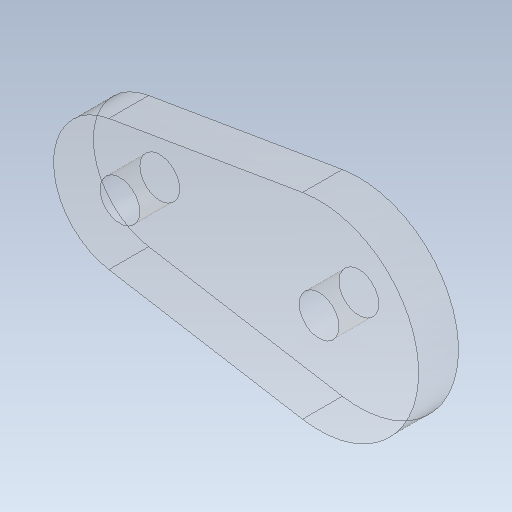
# Autodesk Inventor part: ウイング抑え
Saved by Autodesk Inventor 2020 (Build 240168000, 168)
## iProperties
Created: 2019-11-29
Part Number: ウイング抑え
Material: ポリカーボネート、クリア
Document SubType Name: Modeling
Designer: tanjihayato
Density: 1.2 g/cm^3
Appearance: ポリカーボネート - クリア
Mass: 1.09296 g
Surface Area: 8.72812 cm^2
Volume: 0.910801 cm^3
Author: tanjihayato
Autodesk Inventor part; units mm, degrees
ref_plane "YZ Plane" through (0, 0, 0) normal (1, 0, 0) x (0, 1, 0)
ref_plane "XZ Plane" through (0, 0, 0) normal (0, 1, 0) x (-1, 0, 0)
ref_plane "XY Plane" through (0, 0, 0) normal (0, 0, 1) x (1, 0, 0)
sketch "スケッチ1" plane through (0, 0, 0) normal (0, 0, 1) x (1, 0, 0)
  circle A0 centre (0, 0) radius 1.5
  circle A1 centre (15, 0) radius 1.5
  arc A2 (-0.8333, 4.9301) -> (-0.8333, -4.9301) centre (0, 0) ccw
  arc A3 (13.75, -7.3951) -> (13.75, 7.3951) centre (15, 0) ccw
  line L0 (-0.8333, 4.9301) -> (13.75, 7.3951)
  line L1 (-0.8333, -4.9301) -> (13.75, -7.3951)
  dimension "d0" = 3
  dimension "d1" = 3
  dimension "d2" = 15
  dimension "d3" = 10
  dimension "d4" = 15
  constraints: 4 centre point, 4 end point, 4 point on circle, 4 tangent, 3 coincident, 1 horizontal alignment
  measures "d0" diameter of A0
  measures "d1" diameter of A1
  measures "d2" distance of A1.centre point (0, 0)
  measures "d3" diameter of A2
  measures "d4" diameter of A3
extrude "押し出し1" add sketch "スケッチ1" along normal blind 3
